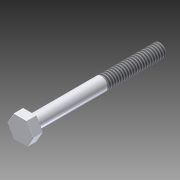
# Autodesk Inventor part: Deck_Bolt
Saved by Autodesk Inventor 2011 SP1 (Build 150282100, 282)
## iProperties
Created: 2011-06-12
Part Number: Deck_Bolt
Document SubType Name: Modeling
Designer: Andrew G. Meyer
Mass: 2.51926 g
Surface Area: 16.5553 cm^2
Volume: 2.51926 cm^3
Density: 1 g/cm^3
Author: Andrew G. Meyer
Autodesk Inventor part; units mm, degrees
ref_plane "YZ Plane" through (0, 0, 0) normal (1, 0, 0) x (0, 1, 0)
ref_plane "XZ Plane" through (0, 0, 0) normal (0, 1, 0) x (-1, 0, 0)
ref_plane "XY Plane" through (0, 0, 0) normal (0, 0, 1) x (1, 0, 0)
sketch "Sketch1" plane through (0, 0, 0) normal (0, 0, 1) x (1, 0, 0)
  circle A0 centre (0, 0) radius 3.175
  dimension "d0" = 6.35
  constraints: 1 centre point, 1 coincident
  measures "d0" diameter of A0
extrude "Extrusion1" add sketch "Sketch1" along normal blind 63.5
sketch "Sketch2" plane through (0, 0, 63.5) normal (0, 0, 1) x (1, 0, 0)
  circle A0 centre (0, 0) radius 3.175 projected
  line L0 (3.2079, 5.5562) -> (6.4158, 0)
  line L1 (6.4158, 0) -> (3.2079, -5.5562)
  line L2 (3.2079, -5.5562) -> (-3.2079, -5.5562)
  line L3 (-3.2079, -5.5562) -> (-6.4158, 0)
  line L4 (-6.4158, 0) -> (-3.2079, 5.5562)
  line L5 (-3.2079, 5.5562) -> (3.2079, 5.5562)
  dimension "d4" = 11.1125
  constraints: 12 end point, 1 coincident, 1 horizontal, 13 other
  measures "d4" distance between parallel lines of L2 L5
extrude "Extrusion2" add sketch "Sketch2" along normal blind 4.7625 contours A0 | L0 L1 L2 L3 L4 L5
fillet "Fillet1" radius 0.254 12 edges at (4.8119, 2.7781, 68.2625) (0, 5.5562, 68.2625) (-4.8119, 2.7781, 68.2625) (-4.8119, -2.7781, 68.2625) (0, -5.5562, 68.2625) (4.8119, -2.7781, 68.2625) (4.8119, -2.7781, 63.5) (4.8119, 2.7781, 63.5) (0, 5.5562, 63.5) (-4.8119, 2.7781, 63.5) (-4.8119, -2.7781, 63.5) (0, -5.5562, 63.5)
thread "Thread1" size "1/4-20 UNC" class "2A" standard "ANSI Unified Screw Threads" length 28.575
body "Solid1"
